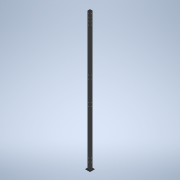
# Autodesk Inventor part: metal supporter
Saved by Autodesk Inventor 2020 (Build 240168000, 168)
## iProperties
Created: 2020-06-26
Part Number: metal supporter
Material: Generic
Document SubType Name: Modeling
Designer: Abbas
Density: 1 g/cm^3
Appearance: Default
Author: Abbas
Autodesk Inventor part; units mm, degrees
ref_plane "YZ Plane" through (0, 0, 0) normal (1, 0, 0) x (0, 1, 0)
ref_plane "XZ Plane" through (0, 0, 0) normal (0, 1, 0) x (-1, 0, 0)
ref_plane "XY Plane" through (0, 0, 0) normal (0, 0, 1) x (1, 0, 0)
sketch "Sketch1" plane through (0, 0, 0) normal (0, 1, 0) x (-1, 0, 0)
  line L0 (15, 20) -> (-15, 20)
  line L1 (-20, 15) -> (-20, -15)
  line L2 (-15, -20) -> (15, -20)
  line L3 (20, -15) -> (20, 15)
  line L4 (20, 20) -> (-20, -20) construction
  line L5 (-20, 20) -> (20, -20) construction
  line L6 (13, 18) -> (-13, 18)
  line L7 (-18, 13) -> (-18, -13)
  line L8 (-13, -18) -> (13, -18)
  line L9 (18, -13) -> (18, 13)
  line L10 (18, 18) -> (-18, -18) construction
  line L11 (-18, 18) -> (18, -18) construction
  line L12 (35, 35) -> (-35, 35)
  line L13 (-35, 35) -> (-35, -35)
  line L14 (-35, -35) -> (35, -35)
  line L15 (35, -35) -> (35, 35)
  line L16 (35, 35) -> (-35, -35) construction
  line L17 (-35, 35) -> (35, -35) construction
  arc A0 (20, 15) -> (15, 20) centre (15, 15) ccw
  arc A1 (18, 13) -> (13, 18) centre (13, 13) ccw
  arc A2 (13, -18) -> (18, -13) centre (13, -13) ccw
  arc A3 (15, -20) -> (20, -15) centre (15, -15) ccw
  arc A4 (-13, 18) -> (-18, 13) centre (-13, 13) ccw
  arc A5 (-15, 20) -> (-20, 15) centre (-15, 15) ccw
  arc A6 (-20, -15) -> (-15, -20) centre (-15, -15) ccw
  arc A7 (-18, -13) -> (-13, -18) centre (-13, -13) ccw
  point P0 (0, 0)
  dimension "d0" = 40
  dimension "d1" = 40
  dimension "d2" = 36
  dimension "d3" = 36
  dimension "d4" = 70
  dimension "d5" = 70
  dimension "d6" = 5
  constraints: 36 end point, 16 point on circle, 16 point on line, 16 tangent, 8 centre point, 7 equal radius, 6 midpoint, 6 parallel, 3 horizontal, 3 perpendicular
  measures "d0" distance of L5.end L4.end
  measures "d1" distance of L4.end L5.start
  measures "d2" distance of L11.end L10.end
  measures "d3" distance of L10.end L11.start
  measures "d4" distance of L14.end L13.end
  measures "d5" distance of L13.end L12.end
  measures "d6" radius of A0
extrude "Extrusion1" add sketch "Sketch1" along normal blind 3 contours L15 L14 L13 L12
extrude "Extrusion2" add sketch "Sketch1" along normal blind 2000 contours A0 L3 A3 L2 A6 L1 A5 L0
sketch "Sketch2" plane through (20, 3, -15) normal (1, 0, 0) x (0, 0, -1)
  line L0 (-30, 0) -> (-30, 1997) projected
  line L1 (-30, 1997) -> (0, 1997) projected
  point P0 (-15, -3)
  point P1 (-15, 1197)
  point P2 (-15, 1147)
  dimension "d18" = 50
  dimension "d19" = 15
  dimension "d20" = 15
  dimension "d21" = 800
  measures "d18" distance of point (-15, 1147) point (-15, 1197)
  measures "d19" distance from line of L0 point (-15, 1197)
  measures "d20" distance from line of L0 point (-15, 1147)
  measures "d21" distance from line of L1 point (-15, 1197)
hole "Hole1" at (20, 1200, 0) at (20, 1150, 0) direction (-1, 0, 0) diameter 8 end through all
sketch "Sketch3" plane through (15, 3, 20) normal (0, 0, 1) x (1, 0, 0)
  line L0 (-30, 0) -> (-30, 1997) projected
  line L1 (-30, 1997) -> (0, 1997) projected
  point P0 (-15, -3)
  point P1 (-15, 1197)
  point P2 (-15, 1147)
  dimension "d29" = 50
  dimension "d30" = 15
  dimension "d31" = 15
  dimension "d32" = 800
  measures "d29" distance of point (-15, 1147) point (-15, 1197)
  measures "d30" distance from line of L0 point (-15, 1197)
  measures "d31" distance from line of L0 point (-15, 1147)
  measures "d32" distance from line of L1 point (-15, 1197)
hole "Hole2" at (0, 1200, 20) at (0, 1150, 20) direction (0, 0, -1) diameter 8 end through all
sketch "Sketch4" plane through (20, 3, -15) normal (1, 0, 0) x (0, 0, -1)
  line L0 (-30, 0) -> (-30, 1997) projected
  line L1 (0, 0) -> (-30, 0) projected
  point P0 (-15, -3)
  point P1 (-15, 150)
  point P2 (-15, 100)
  dimension "d40" = 50
  dimension "d41" = 15
  dimension "d42" = 15
  dimension "d43" = 100
  measures "d40" distance of point (-15, 100) point (-15, 150)
  measures "d41" distance from line of L0 point (-15, 150)
  measures "d42" distance from line of L0 point (-15, 100)
  measures "d43" distance from line of L1 point (-15, 100)
hole "Hole3" at (20, 153, 0) at (20, 103, 0) direction (-1, 0, 0) diameter 8 end through all
sketch "Sketch5" plane through (15, 3, 20) normal (0, 0, 1) x (1, 0, 0)
  line L0 (0, 0) -> (0, 1997) projected
  line L1 (0, 0) -> (-30, 0) projected
  point P0 (-15, -3)
  point P1 (-15, 150)
  point P2 (-15, 100)
  dimension "d51" = 50
  dimension "d52" = 15
  dimension "d53" = 15
  dimension "d54" = 100
  measures "d51" distance of point (-15, 100) point (-15, 150)
  measures "d52" distance from line of L0 point (-15, 150)
  measures "d53" distance from line of L0 point (-15, 100)
  measures "d54" distance from line of L1 point (-15, 100)
hole "Hole4" at (0, 153, 20) at (0, 103, 20) direction (0, 0, -1) diameter 8 end through all
sketch "Sketch6" plane through (15, 3, 20) normal (0, 0, 1) x (1, 0, 0)
  line L0 (-30, 1997) -> (0, 1997) projected
  line L1 (-30, 0) -> (-30, 1997) projected
  point P0 (-15, -3)
  point P1 (-15, 1972)
  point P2 (-15, 1922)
  dimension "d62" = 50
  dimension "d63" = 25
  dimension "d64" = 15
  dimension "d65" = 15
  measures "d62" distance of point (-15, 1922) point (-15, 1972)
  measures "d63" distance from line of L0 point (-15, 1972)
  measures "d64" distance from line of L1 point (-15, 1972)
  measures "d65" distance from line of L1 point (-15, 1922)
hole "Hole5" at (0, 1975, 20) at (0, 1925, 20) direction (0, 0, -1) diameter 8 end through all
sketch "Sketch7" plane through (20, 3, -15) normal (1, 0, 0) x (0, 0, -1)
  line L0 (-30, 1997) -> (0, 1997) projected
  line L1 (-30, 0) -> (-30, 1997) projected
  point P0 (-15, -3)
  point P1 (-15, 1972)
  point P2 (-15, 1922)
  dimension "d73" = 25
  dimension "d74" = 50
  dimension "d75" = 15
  dimension "d76" = 15
  measures "d73" distance from line of L0 point (-15, 1972)
  measures "d74" distance of point (-15, 1972) point (-15, 1922)
  measures "d75" distance from line of L1 point (-15, 1972)
  measures "d76" distance from line of L1 point (-15, 1922)
hole "Hole6" at (20, 1975, 0) at (20, 1925, 0) direction (-1, 0, 0) diameter 8 end through all
sketch "Sketch9" plane through (20, 3, -15) normal (1, 0, 0) x (0, 0, -1)
  line L0 (0, 0) -> (0, 1997) projected
  circle A0 centre (-15, 1147) radius 4 projected
  point P0 (-15, -3)
  point P1 (-15, 847)
  point P2 (-15, 797)
  dimension "d95" = 50
  dimension "d96" = 15
  dimension "d97" = 15
  dimension "d98" = 300
  measures "d95" distance of point (-15, 797) point (-15, 847)
  measures "d96" distance from line of L0 point (-15, 847)
  measures "d97" distance from line of L0 point (-15, 797)
  measures "d98" distance of A0.centre point (-15, 847)
hole "Hole8" at (20, 850, 0) at (20, 800, 0) direction (-1, 0, 0) diameter 8 end through all
sketch "Sketch10" plane through (15, 3, 20) normal (0, 0, 1) x (1, 0, 0)
  line L0 (0, 0) -> (0, 1997) projected
  circle A0 centre (-15, 1147) radius 4 projected
  point P0 (-15, -3)
  point P1 (-15, 847)
  point P2 (-15, 797)
  dimension "d106" = 50
  dimension "d107" = 15
  dimension "d108" = 15
  dimension "d109" = 300
  measures "d106" distance of point (-15, 797) point (-15, 847)
  measures "d107" distance from line of L0 point (-15, 847)
  measures "d108" distance from line of L0 point (-15, 797)
  measures "d109" distance of A0.centre point (-15, 847)
hole "Hole9" at (0, 850, 20) at (0, 800, 20) direction (0, 0, -1) diameter 8 end through all
sketch "Sketch11" plane through (15, 3, 20) normal (0, 0, 1) x (1, 0, 0)
  line L0 (0, 0) -> (0, 1997) projected
  line L1 (-30, 1997) -> (0, 1997) projected
  point P0 (-15, -3)
  point P1 (-15, 1877)
  point P2 (-15, 1827)
  dimension "d117" = 50
  dimension "d118" = 15
  dimension "d119" = 15
  dimension "d120" = 120
  measures "d117" distance of point (-15, 1827) point (-15, 1877)
  measures "d118" distance from line of L0 point (-15, 1877)
  measures "d119" distance from line of L0 point (-15, 1827)
  measures "d120" distance from line of L1 point (-15, 1877)
hole "Hole10" at (0, 1880, 20) at (0, 1830, 20) direction (0, 0, -1) diameter 8 end through all
sketch "Sketch12" plane through (20, 3, -15) normal (1, 0, 0) x (0, 0, -1)
  line L0 (0, 0) -> (0, 1997) projected
  line L1 (-30, 1997) -> (0, 1997) projected
  point P0 (-15, -3)
  point P1 (-15, 1877)
  point P2 (-15, 1827)
  dimension "d128" = 50
  dimension "d129" = 15
  dimension "d130" = 15
  dimension "d131" = 120
  measures "d128" distance of point (-15, 1827) point (-15, 1877)
  measures "d129" distance from line of L0 point (-15, 1827)
  measures "d130" distance from line of L0 point (-15, 1877)
  measures "d131" distance from line of L1 point (-15, 1877)
hole "Hole11" at (20, 1880, 0) at (20, 1830, 0) direction (-1, 0, 0) diameter 8 end through all
body "Solid1"
